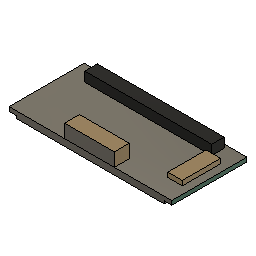
E-Ink 2.13 v3 (Autodesk Fusion 360 design; units mm, degrees)
Autodesk Fusion 360 part; units mm, degrees
sketch "Sketch1" plane through (0, 0, 0) normal (0, 1, 0) x (1, 0, 0)
  line L0 (-32.7, 15.1) -> (32.7, 15.1)
  line L1 (32.7, 15.1) -> (32.7, -15.1)
  line L2 (32.7, -15.1) -> (-32.7, -15.1)
  line L3 (-32.7, -15.1) -> (-32.7, 15.1)
  line L4 (-10.4, -9.1) -> (9.6, -9.1)
  line L5 (9.6, -9.1) -> (9.6, -15.1)
  line L6 (9.6, -15.1) -> (-10.4, -15.1)
  line L7 (-10.4, -15.1) -> (-10.4, -9.1)
  line L8 (-25.95, 13.6) -> (25.05, 13.6)
  line L9 (25.05, 13.6) -> (25.05, 8.6)
  line L10 (25.05, 8.6) -> (-25.95, 8.6)
  line L11 (-25.95, 8.6) -> (-25.95, 13.6)
  line L12 (23.9, 7.5) -> (29.7, 7.5)
  line L13 (29.7, 7.5) -> (29.7, -7.9)
  line L14 (29.7, -7.9) -> (23.9, -7.9)
  line L15 (23.9, -7.9) -> (23.9, 7.5)
  line L16 (-29.6, 15.1) -> (-29.6, -15.1)
  line L17 (29.7, -15.1) -> (29.7, 15.1)
  dimension "d1" = 65.4
  dimension "d2" = 30.2
  dimension "d3" = 32.7
  dimension "d4" = 15.1
  dimension "d5" = 6
  dimension "d6" = 20
  dimension "d7" = 23.1
  dimension "d8" = 5
  dimension "d9" = 51
  dimension "d10" = 7.65
  dimension "d11" = 1.5
  dimension "d12" = 5.8
  dimension "d13" = 15.4
  dimension "d14" = 7.6
  dimension "d15" = 3
  dimension "d16" = 59.3
  dimension "d17" = 3
  constraint horizontal L0
  constraint vertical L1
  constraint horizontal L2
  constraint vertical L3
  constraint horizontal L4
  constraint vertical L5
  constraint horizontal L6
  constraint vertical L7
  constraint coincident L2 L5.end
  constraint horizontal L8
  constraint vertical L9
  constraint horizontal L10
  constraint vertical L11
  constraint horizontal L12
  constraint vertical L13
  constraint horizontal L14
  constraint vertical L15
  constraint coincident L0 L16.start
  constraint coincident L2 L16.end
  constraint perpendicular L2 L16
  constraint coincident L2 L17.start
  constraint coincident L0 L17.end
  constraint perpendicular L0 L17
  measures "d1" distance of L0.start L0.end
  measures "d2" distance of L0.start L2.end
  measures "d3" distance of origin L1
  measures "d4" distance of origin L2
  measures "d5" distance of L4.start L6.end
  measures "d6" distance of L4.start L4.end
  measures "d7" distance of L1 L5
  measures "d8" distance of L8.start L10.end
  measures "d9" distance of L8.start L8.end
  measures "d10" distance of L1 L9
  measures "d11" distance of L0 L8
  measures "d12" distance of L12.start L12.end
  measures "d13" distance of L12 L14
  measures "d14" distance of L0 L12
  measures "d15" distance of L1 L13
  measures "d16" distance of L16 L17
  measures "d17" distance of L1 L17
extrude "Extrude1" add sketch "Sketch1" against normal blind 1.65 contours L0 L2 L3 L16 | L0 L2 L4 L5 L7 L12 L14 L15 L16 L17 | L0 L1 L2 L13 L17 | L12 L13 L14 L15 L17 | L2 L4 L5 L6 L7 | L8 L9 L10 L11 makes body 1
extrude "Extrude2" add sketch "Sketch1" against normal blind 2.7 contours L0 L2 L4 L5 L7 L12 L14 L15 L16 L17 | L12 L13 L14 L15 L17 | L2 L4 L5 L6 L7 | L8 L9 L10 L11 bodies 1
extrude "Extrude3" add sketch "Sketch1" along normal blind 5.4 contours L2 L4 L5 L6 L7 bodies 1
extrude "Extrude4" add sketch "Sketch1" along normal blind 1.9 contours L12 L13 L14 L15 L17 bodies 1
extrude "Extrude5" add sketch "Sketch1" along normal blind 3.9 contours L8 L9 L10 L11 bodies 1
split "Split1" by plane through (0, 0, 0) normal (0, 1, 0) bodies 1 makes body 2 at (27.7667, 1.9, 2.7667) makes body 3 at (2.9333, 5.4, 13.1) makes body 4 at (-8.95, 3.9, -11.9333)
equation "d3 = d1 / 2"
equation "d4 = d2 / 2"
